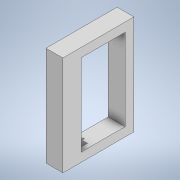
# Autodesk Inventor part: Framuga
Saved by Autodesk Inventor 2020.1 (Build 241239000, 239)
## iProperties
Created: 2022-04-03
Part Number: Framuga
Material: Generic
Document SubType Name: Modeling
Designer: OEM
Density: 1 g/cm^3
Appearance: Default
Author: OEM
Autodesk Inventor part; units mm, degrees
ref_plane "YZ Plane" through (0, 0, 0) normal (1, 0, 0) x (0, 1, 0)
ref_plane "XZ Plane" through (0, 0, 0) normal (0, 1, 0) x (-1, 0, 0)
ref_plane "XY Plane" through (0, 0, 0) normal (0, 0, 1) x (1, 0, 0)
sketch "Sketch2" plane through (0, 0, 0) normal (0, 1, 0) x (-1, 0, 0)
  line L0 (7, 12) -> (-7, 12)
  line L1 (-7, 12) -> (-7, -12)
  line L2 (-7, -12) -> (7, -12)
  line L3 (7, -12) -> (7, 12)
  line L4 (7, 12) -> (-7, -12) construction
  line L5 (-7, 12) -> (7, -12) construction
  line L6 (12, 20.5714) -> (12, -20.5714) construction
  line L7 (-12, -20.5714) -> (-12, 20.5714)
  line L8 (-12, 20.5714) -> (12, -20.5714) construction
  line L9 (12, 20.5714) -> (-12, -20.5714) construction
  line L10 (41, 0) -> (-38, 0) construction
  circle A0 centre (0, -14) radius 1
  line L11 (-7, -12) -> (-7, -29.1429) construction
  circle A1 centre (0, -6) radius 1 construction
  line L12 (7, 12) -> (7, 20.5714)
  line L13 (7, -12) -> (7, -20.5714)
  line L14 (7, 20.5714) -> (-12, 20.5714)
  line L15 (-12, -20.5714) -> (7, -20.5714) construction
  line L16 (7, -20.5714) -> (12, -20.5714) construction
  line L17 (7, 20.5714) -> (12, 20.5714) construction
  line L18 (-12, -20.5714) -> (-12, -59.4286)
  line L19 (0, 40.4504) -> (0, -46.455) construction
  line L20 (7, -20.5714) -> (7, -59.4286)
  line L21 (7, -59.4286) -> (-12, -59.4286)
  line L22 (7, 0) -> (-12, 0)
  line L23 (7, -49.4286) -> (-12, -49.4286)
  line L24 (-7, 12) -> (-7, 20.5714)
  circle A2 centre (0, 14) radius 1
  line L25 (-12, 18) -> (7, 18)
  point P0 (0, 0)
  point P1 (0, 0)
  point P2 (0, 0)
  point P3 (-7, 0)
  point P4 (-7, 18)
  point P5 (0, 0)
  dimension "d0" = 14
  dimension "d1" = 24
  dimension "d2" = 5
  dimension "d3" = 2
  dimension "d4" = 7
  dimension "d5" = 2
  dimension "d6" = 6
  dimension "d7" = 2
  dimension "d11" = 80
  dimension "d26" = 6
  dimension "d27" = 10
  constraints: 52 end point, 14 point on line, 9 midpoint, 5 parallel, 4 perpendicular, 3 centre point, 3 horizontal, 2 vertical, 1 collinear, 1 symmetric about line, 2 other
  measures "d0" distance of L1.end L2.end
  measures "d1" distance of L2.end L0.start
  measures "d2" distance between parallel lines of L6 L3
  measures "d3" diameter of A0
  measures "d4" distance from line of L11 A0.centre
  measures "d5" distance from line of L2 A0.centre
  measures "d6" distance from line of L2 A1.centre
  measures "d7" diameter of A1
  measures "d11" distance between parallel lines of L21 L14
  measures "d26" distance between parallel lines of L0 L25
  measures "d27" distance between parallel lines of L21 L23
extrude "Extrusion1" add sketch "Sketch2" against normal blind 10 contours L0 L24 L25 L12 | L1 L22 L7 L25 L24 | L25 L24 L14 L12 | L1 L2 L13 L20 L23 L18 L7 L22 | L25 L7 L14 L24 | L20 L21 L18 L23
extrude "Extrusion2" add sketch "Sketch2" along normal blind 102 contours L3 L22 L1 L0 | L0 L24 L25 L12 | L1 L22 L7 L25 L24 | L3 L2 L1 L22 | L25 L24 L14 L12 | L1 L2 L13 L20 L23 L18 L7 L22 | L25 L7 L14 L24 | L20 L21 L18 L23 | A0 | A2
extrude "Extrusion3" cut sketch "Sketch2" along normal blind 92 contours L3 L2 L1 L22 | L1 L2 L13 L20 L23 L18 L7 L22 | A0
extrude "Extrusion4" cut sketch "Sketch2" along normal blind 20 contours L3 L22 L1 L0 | L0 L24 L25 L12 | A2
body "Solid1"
